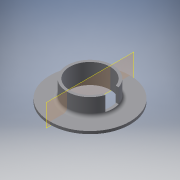
# Autodesk Inventor part: customWasher
Saved by Autodesk Inventor 2019.3 (Build 233278000, 278)
## iProperties
Created: 2019-04-09
Part Number: customWasher
Material: Generic
Document SubType Name: Modeling
Designer: steele
Density: 1 g/cm^3
Appearance: Default
Author: steele
Autodesk Inventor part; units mm, degrees
ref_plane "YZ Plane" through (0, 0, 0) normal (1, 0, 0) x (0, 1, 0)
ref_plane "XZ Plane" through (0, 0, 0) normal (0, 1, 0) x (-1, 0, 0)
ref_plane "XY Plane" through (0, 0, 0) normal (0, 0, 1) x (1, 0, 0)
sketch "Sketch1" plane through (0, 0, 0) normal (0, 0, 1) x (1, 0, 0)
  line L0 (21.844, 0) -> (21.844, -12.7)
  line L1 (25.019, -15.875) -> (38.1, -15.875)
  line L2 (38.1, -15.875) -> (38.1, -18.415)
  line L3 (38.1, -18.415) -> (19.304, -18.415)
  line L4 (19.304, -18.415) -> (19.304, 0)
  line L5 (19.304, 0) -> (21.844, 0)
  line L6 (0, 0) -> (27.9096, 0) construction
  arc A0 (21.844, -12.7) -> (25.019, -15.875) centre (25.019, -12.7) ccw
  line L7 (0, 0) -> (0, -18.415) construction
  dimension "d0" = 19.304
  dimension "d1" = 18.415
  dimension "d2" = 2.54
  dimension "d3" = 2.54
  dimension "d5" = 3.175
  dimension "d9" = 38.1
  constraints: 16 end point, 4 perpendicular, 2 horizontal, 2 point on circle, 2 tangent, 1 centre point, 1 collinear, 1 point on line
  measures "d0" distance from line of L6.start L4
  measures "d1" distance between parallel lines of L3 L5
  measures "d2" distance between parallel lines of L0 L4
  measures "d3" distance between parallel lines of L3 L1
  measures "d5" radius of A0
  measures "d9" distance between parallel lines of L2 L7
revolve "Revolution1" add sketch "Sketch1" angle 360 about axis through (0, 0, 0) along (0, -1, 0)
sketch "Sketch2" plane through (0, 0, 0) normal (1, 0, 0) x (0, 1, 0)
  line L0 (0, 0) -> (-26.67, 0) construction
  line L1 (-13.97, -6.35) -> (0, -6.35)
  line L2 (0, -6.35) -> (0, 6.35)
  line L3 (0, 6.35) -> (-13.97, 6.35)
  line L4 (-13.97, 6.35) -> (-13.97, -6.35)
  line L5 (-13.97, -6.35) -> (0, 6.35) construction
  line L6 (0, -6.35) -> (-13.97, 6.35) construction
  line L7 (0, 19.304) -> (0, -19.304) projected
  point P0 (-6.985, 0)
  dimension "d10" = 12.7
  dimension "d11" = 13.97
  dimension "d12" = 0
  constraints: 14 end point, 2 horizontal, 2 midpoint, 2 parallel, 1 perpendicular, 1 point on line
  measures "d10" distance of L1.end L2.end
  measures "d11" distance of L2.end L3.end
  measures "d12" distance between parallel lines of L7 L2
extrude "Extrusion1" cut sketch "Sketch2" along normal blind 22.86
body "Solid1"
